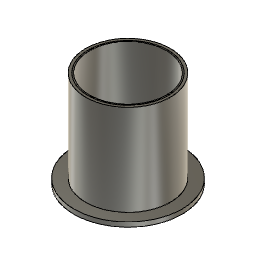
ergotron-lx-sleeve v4 (Autodesk Fusion 360 design; units mm, degrees)
Autodesk Fusion 360 part; units mm, degrees
sketch "Sketch1" plane through (0, 0, 0) normal (0, 0, 1) x (1, 0, 0)
  circle A0 centre (0, 0) radius 17.45
  circle A1 centre (0, 0) radius 18.6
  circle A2 centre (0, 0) radius 23.75
  dimension "d1" = 34.9
  dimension "d2" = 37.2
  dimension "d3" = 47.5
  constraint coincident A0.centre A1.centre
  constraint concentric A0 A2
  measures "d1" diameter of A0
  measures "d2" diameter of A1
  measures "d3" diameter of A2
extrude "Extrude1" add sketch "Sketch1" along normal blind 42 contours A1 makes body 1
extrude "Extrude2" add sketch "Sketch1" along normal blind 2 contours A2 bodies 1
sketch "Sketch1 (2)" plane through (0, 0, 0) normal (0, 0, 1) x (1, 0, 0) in component "pipe-added-ID"
  circle A0 centre (0, 0) radius 16.9
  circle A1 centre (0, 0) radius 17.45
  circle A2 centre (0, 0) radius 18.6
  circle A3 centre (0, 0) radius 17.45
  dimension "d8" = 33.8
  constraint coincident A0.centre A1.centre
  constraint concentric A1 A3
  measures "d8" diameter of A0
extrude "Extrude1'" add sketch "Sketch1 (2)" along normal up to surface (42 mm away) separate body contours A1 A3 makes body 2 in component "pipe-added-ID"
component "pipe-added-ID" placed x (1, 0, 0) y (0, 1, 0) z (0, 0, 1) at (0, 0, 0)
